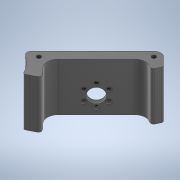
# Autodesk Inventor part: left_motor_short
Saved by Autodesk Inventor 2020 (Build 240168000, 168)
## iProperties
Created: 2023-12-16
Part Number: left_motor_short
Material: Пластмасса, непрозрачная, черная
Document SubType Name: Modeling
Designer: denis
Density: 0.952 g/cm^3
Appearance: Гладкая — черная
Author: denis
## iProperties of the stored document _3DПЕЧАТЬ.ipt
Created: 2024-02-21
Part Number: _3DПЕЧАТЬ
Material: Типовые
Document SubType Name: Modeling
Designer: 4s
Density: 1 g/cm^3
Appearance: По умолчанию
Author: 4s
Autodesk Inventor part; units mm, degrees
ref_plane "YZ Plane" through (0, 0, 0) normal (1, 0, 0) x (0, 1, 0)
ref_plane "XZ Plane" through (0, 0, 0) normal (0, 1, 0) x (-1, 0, 0)
ref_plane "XY Plane" through (0, 0, 0) normal (0, 0, 1) x (1, 0, 0)
sketch "Эскиз1" plane through (0, 0, 0) normal (0, 1, 0) x (-1, 0, 0)
  line L0 (34.2947, -76.014) -> (76.014, -34.2947)
  arc A0 (83.085, -34.2947) -> (76.014, -34.2947) centre (79.5495, -37.8302) ccw
  line L1 (83.085, -34.2947) -> (87.156, -38.3657)
  line L2 (46.3155, -73.8927) -> (73.8927, -46.3155)
  arc A1 (85.2064, -46.3155) -> (73.8927, -46.3155) centre (79.5495, -51.9723) ccw
  line L3 (85.2064, -46.3155) -> (87.5645, -48.6736)
  line L4 (92.5543, -49.5852) -> (94.5192, -45.7288)
  line L5 (87.156, -38.3657) -> (94.5192, -45.7288)
  line L6 (34.2947, -83.085) -> (38.3657, -87.156)
  arc A2 (34.2947, -76.014) -> (34.2947, -83.085) centre (37.8302, -79.5495) ccw
  arc A3 (46.3155, -73.8927) -> (46.3155, -85.2064) centre (51.9723, -79.5495) ccw
  line L7 (48.6736, -87.5645) -> (46.3155, -85.2064)
  line L8 (48.7014, -93.0224) -> (45.7288, -94.5192)
  line L9 (38.3657, -87.156) -> (45.7288, -94.5192)
  spline S0 degree 4 poles (87.5645, -48.6736) (88.1327, -49.2418) (88.8708, -49.8865) (89.7495, -50.471) (90.7127, -50.7263) (91.4939, -50.6999) (92.0261, -50.3682) (92.3519, -49.9478) (92.5543, -49.5852) knots 0 0 0 0 0 0.3763 0.501335 0.614666 0.722287 1 1 1 1 1
  spline S1 degree 4 poles (48.6736, -87.5645) (49.2196, -88.1111) (49.8318, -88.8375) (50.3553, -89.7359) (50.492, -90.7638) (50.3179, -91.6771) (49.7988, -92.3195) (49.2087, -92.7429) (48.7014, -93.0224) knots 0 0 0 0 0 0.349502 0.469309 0.582088 0.694155 1 1 1 1 1
  line L10 (-34.2947, -83.085) -> (-38.3657, -87.156)
  arc A4 (-34.2947, -83.085) -> (-34.2947, -76.014) centre (-37.8302, -79.5495) ccw
  line L11 (-34.2947, -76.014) -> (-76.014, -34.2947)
  arc A5 (-76.014, -34.2947) -> (-83.085, -34.2947) centre (-79.5495, -37.8302) ccw
  line L12 (-83.085, -34.2947) -> (-87.156, -38.3657)
  spline S2 degree 4 poles (-87.5645, -48.6736) (-88.2874, -48.92) (-89.2024, -49.1688) (-90.211, -49.3633) (-91.1746, -49.4987) (-91.8001, -49.5729) (-92.1944, -49.6036) (-92.4378, -49.611) (-92.5543, -49.5852) knots 0 0 0 0 0 0.417996 0.557878 0.680942 0.788351 1 1 1 1 1
  line L13 (-85.2064, -46.3155) -> (-87.5645, -48.6736)
  arc A6 (-73.8927, -46.3155) -> (-85.2064, -46.3155) centre (-79.5495, -51.9723) ccw
  line L14 (-46.3155, -73.8927) -> (-73.8927, -46.3155)
  arc A7 (-46.3155, -85.2064) -> (-46.3155, -73.8927) centre (-51.9723, -79.5495) ccw
  spline S3 degree 4 poles (-48.6736, -87.5645) (-49.2196, -88.1111) (-49.8318, -88.8375) (-50.3553, -89.7359) (-50.492, -90.7638) (-50.3179, -91.6771) (-49.7988, -92.3195) (-49.2087, -92.7429) (-48.7014, -93.0224) knots 0 0 0 0 0 0.349502 0.469309 0.582088 0.694155 1 1 1 1 1
  line L15 (-48.6736, -87.5645) -> (-46.3155, -85.2064)
  arc A8 (-92.5543, 49.5852) -> (-92.5543, -49.5852) centre (0, 0) ccw construction
  arc A9 (-48.7014, -93.0224) -> (48.7014, -93.0224) centre (0, 0) ccw construction
  line L16 (-38.3657, -87.156) -> (-45.7288, -94.5192)
  line L17 (-87.156, -38.3657) -> (-94.5192, -45.7288)
  line L18 (-92.5543, -49.5852) -> (-94.5192, -45.7288)
  line L19 (-48.7014, -93.0224) -> (-45.7288, -94.5192)
  line L20 (0, 0) -> (0, 95.3237) construction
  line L21 (34.2947, -76.014) -> (76.014, -34.2947)
  arc A10 (83.085, -34.2947) -> (76.014, -34.2947) centre (79.5495, -37.8302) ccw
  line L22 (83.085, -34.2947) -> (87.156, -38.3657)
  line L23 (46.3155, -73.8927) -> (73.8927, -46.3155)
  arc A11 (85.2064, -46.3155) -> (73.8927, -46.3155) centre (79.5495, -51.9723) ccw
  line L24 (85.2064, -46.3155) -> (87.5645, -48.6736)
  line L25 (92.5543, -49.5852) -> (94.5192, -45.7288)
  arc A12 (92.5543, -49.5852) -> (92.5543, 49.5852) centre (0, 0) ccw construction
  line L26 (87.156, -38.3657) -> (94.5192, -45.7288)
  line L27 (34.2947, -83.085) -> (38.3657, -87.156)
  arc A13 (34.2947, -76.014) -> (34.2947, -83.085) centre (37.8302, -79.5495) ccw
  arc A14 (46.3155, -73.8927) -> (46.3155, -85.2064) centre (51.9723, -79.5495) ccw
  line L28 (48.6736, -87.5645) -> (46.3155, -85.2064)
  line L29 (48.7014, -93.0224) -> (45.7288, -94.5192)
  line L30 (38.3657, -87.156) -> (45.7288, -94.5192)
  arc A15 (-48.7014, -93.0224) -> (48.7014, -93.0224) centre (0, 0) ccw construction
  spline S4 degree 4 poles (87.5645, -48.6736) (88.1327, -49.2418) (88.8708, -49.8865) (89.7495, -50.471) (90.7127, -50.7263) (91.4939, -50.6999) (92.0261, -50.3682) (92.3519, -49.9478) (92.5543, -49.5852) knots 0 0 0 0 0 0.3763 0.501335 0.614666 0.722287 1 1 1 1 1
  spline S5 degree 4 poles (48.6736, -87.5645) (49.2196, -88.1111) (49.8318, -88.8375) (50.3553, -89.7359) (50.492, -90.7638) (50.3179, -91.6771) (49.7988, -92.3195) (49.2087, -92.7429) (48.7014, -93.0224) knots 0 0 0 0 0 0.349502 0.469309 0.582088 0.694155 1 1 1 1 1
  line L31 (52.2091, 91.1) -> (48.6736, 87.5645) construction
  line L32 (52.2091, 91.1) -> (48.6736, 87.5645) construction
  line L33 (48.6736, 87.5645) -> (52.2091, 91.1) construction
  spline S6 degree 2 poles (48.6736, 87.5645) (52.2091, 91.1) (48.7014, 93.0224) knots 1 1 1 2 2 2 construction
  line L34 (52.2091, 91.1) -> (48.7014, 93.0224) construction
  line L35 (91.1, 52.2091) -> (52.2091, 91.1) construction
  arc A16 (92.5543, 49.5852) -> (48.7014, 93.0224) centre (0, 0) ccw construction
  line L36 (44.1942, 76.014) -> (76.014, 44.1942) construction
  line L37 (0, 56.6418) -> (-35.5516, 86.4744) construction
  arc A17 (0, 67.941) -> (23.7825, 76.5969) centre (0, 104.941) ccw construction
  arc A18 (-23.7825, 76.5969) -> (0, 67.941) centre (0, 104.941) ccw construction
  line L38 (-23.7825, 76.5969) -> (-35.2734, 86.2384) construction
  line L39 (0, 104.941) -> (-23.6028, 54.3247) construction
  arc A19 (-28.0199, 71.0163) -> (5.5413, 61.2914) centre (0, 104.941) ccw construction
  arc A20 (5.5413, 61.2914) -> (28.0199, 71.0163) centre (0, 104.941) ccw construction
  arc A21 (-30.6393, 73.2144) -> (-37.3889, 72.9198) centre (-33.8534, 69.3842) ccw construction
  line L40 (0, 56.6418) -> (23.7825, 76.5969) construction
  line L41 (23.7825, 76.5969) -> (35.2734, 86.2384) construction
  line L42 (0, 0) -> (74.2462, 74.2462) construction
  line L43 (42.6652, 95.941) -> (42.0492, 94.5734) construction
  line L44 (42.0492, 94.5734) -> (42.6652, 95.941) construction
  spline S7 degree 2 poles (42.0492, 94.5734) (42.6652, 95.941) (43.577, 95.5303) knots 1 1 1 2 2 2 construction
  line L45 (42.6652, 95.941) -> (43.577, 95.5303) construction
  arc A22 (-44.1942, 76.014) -> (-44.1942, 83.085) centre (-47.7297, 79.5495) ccw construction
  arc A23 (92.5543, -49.5852) -> (92.5543, 49.5852) centre (0, 0) ccw construction
  circle A24 centre (0, 0) radius 35 construction
  spline S8 degree 2 poles (-48.6736, 87.5645) (-52.2091, 91.1) (-48.7014, 93.0224) knots 1 1 1 2 2 2 construction
  line L46 (-48.6736, 87.5645) -> (-52.2091, 91.1) construction
  line L47 (-52.2091, 91.1) -> (-48.7014, 93.0224) construction
  arc A25 (-83.085, 44.1942) -> (-76.014, 44.1942) centre (-79.5495, 47.7297) ccw construction
  line L48 (-83.085, 44.1942) -> (-85.2064, 46.3155) construction
  line L49 (-44.1942, 76.014) -> (-46.3155, 73.8927) construction
  arc A26 (-48.7014, 93.0224) -> (-92.5543, 49.5852) centre (0, 0) ccw construction
  line L50 (-42.6652, 95.941) -> (-42.0492, 94.5734) construction
  arc A27 (-43.577, 95.5303) -> (-48.7014, 93.0224) centre (0, 0) ccw
  ellipse E0 centre (0, 102.7511) end of major axis (-44.5159, 105.2445) minor radius 28.887 (-42.0492, 94.5734) -> (-35.2734, 86.2384) ccw
  line L51 (-42.0492, 94.5734) -> (-42.6652, 95.941) construction
  spline S9 degree 2 poles (-42.0492, 94.5734) (-42.6652, 95.941) (-43.577, 95.5303) knots 1 1 1 2 2 2 construction
  line L52 (-42.6652, 95.941) -> (-43.577, 95.5303) construction
  line L53 (-42.0492, 94.5734) -> (-42.6652, 95.941) construction
  spline S10 degree 2 poles (-42.0492, 94.5734) (-42.6652, 95.941) (-43.577, 95.5303) knots 1 1 1 2 2 2
  line L54 (-42.6652, 95.941) -> (-43.577, 95.5303) construction
  line L55 (-42.6652, 95.941) -> (-43.577, 95.5303) construction
  line L56 (-44.1942, 83.085) -> (-48.6736, 87.5645) construction
  line L57 (-37.3889, 72.9198) -> (-76.014, 34.2947)
  arc A28 (-83.085, 34.2947) -> (-76.014, 34.2947) centre (-79.5495, 37.8302) ccw
  line L58 (-83.085, 34.2947) -> (-90.6891, 41.8987)
  arc A29 (-87.3563, 48.4654) -> (-90.6891, 41.8987) centre (0, 0) ccw construction
  line L59 (-93.5297, 47.6709) -> (-92.5543, 49.5852) construction
  arc A30 (85.2064, -46.3155) -> (73.8927, -46.3155) centre (79.5495, -51.9723) ccw construction
  line L60 (85.2064, -46.3155) -> (87.5645, -48.6736) construction
  spline S11 degree 2 poles (87.5645, -48.6736) (91.1, -52.2091) (92.5543, -49.5852) knots 1 1 1 2 2 2 construction
  line L61 (87.5645, -48.6736) -> (91.1, -52.2091) construction
  line L62 (91.1, -52.2091) -> (92.5543, -49.5852) construction
  line L63 (46.3155, -73.8927) -> (73.8927, -46.3155) construction
  line L64 (48.6736, -87.5645) -> (46.3155, -85.2064) construction
  line L65 (48.6736, -87.5645) -> (52.2091, -91.1) construction
  spline S12 degree 2 poles (48.6736, -87.5645) (52.2091, -91.1) (48.7014, -93.0224) knots 1 1 1 2 2 2 construction
  line L66 (52.2091, -91.1) -> (48.7014, -93.0224) construction
  arc A31 (46.3155, -73.8927) -> (46.3155, -85.2064) centre (51.9723, -79.5495) ccw construction
  arc A32 (48.7014, -93.0224) -> (92.5543, -49.5852) centre (0, 0) ccw construction
  arc A33 (-48.7014, -93.0224) -> (48.7014, -93.0224) centre (0, 0) ccw construction
  arc A34 (-90.6891, 41.8987) -> (-87.3563, 48.4654) centre (0, 0) ccw construction
  line L67 (42.6652, 95.941) -> (-42.6652, 95.941) construction
  line L68 (-48.6736, -87.5645) -> (-52.2091, -91.1) construction
  spline S13 degree 2 poles (-48.6736, -87.5645) (-52.2091, -91.1) (-48.7014, -93.0224) knots 1 1 1 2 2 2 construction
  line L69 (-52.2091, -91.1) -> (-48.7014, -93.0224) construction
  line L70 (-91.1, -52.2091) -> (-92.5543, -49.5852) construction
  spline S14 degree 2 poles (-87.5645, -48.6736) (-91.1, -52.2091) (-92.5543, -49.5852) knots 1 1 1 2 2 2 construction
  line L71 (-87.5645, -48.6736) -> (-91.1, -52.2091) construction
  arc A35 (-92.5543, -49.5852) -> (-48.7014, -93.0224) centre (0, 0) ccw construction
  line L72 (-48.6736, -87.5645) -> (-46.3155, -85.2064) construction
  arc A36 (-73.8927, -46.3155) -> (-85.2064, -46.3155) centre (-79.5495, -51.9723) ccw construction
  line L73 (-85.2064, -46.3155) -> (-87.5645, -48.6736) construction
  line L74 (-46.3155, -73.8927) -> (-73.8927, -46.3155) construction
  arc A37 (-46.3155, -85.2064) -> (-46.3155, -73.8927) centre (-51.9723, -79.5495) ccw construction
  arc A38 (-92.5543, 49.5852) -> (-92.5543, -49.5852) centre (0, 0) ccw construction
  arc A39 (44.1942, 83.085) -> (44.1942, 76.014) centre (47.7297, 79.5495) ccw construction
  arc A40 (44.0271, 95.3237) -> (43.577, 95.5303) centre (0, 0) ccw construction
  line L75 (42.6652, 95.941) -> (43.577, 95.5303) construction
  arc A41 (48.7014, 93.0224) -> (44.0271, 95.3237) centre (0, 0) ccw construction
  line L76 (52.2091, 91.1) -> (48.7014, 93.0224) construction
  line L77 (83.085, 44.1942) -> (87.5645, 48.6736) construction
  ellipse E1 centre (0, 102.7511) end of major axis (44.5159, 105.2445) minor radius 28.887 (35.2734, 86.2384) -> (42.0492, 94.5734) ccw construction
  arc A42 (76.014, 44.1942) -> (83.085, 44.1942) centre (79.5495, 47.7297) ccw construction
  line L78 (0, 0) -> (0, 209.8821) construction
  arc A43 (43.577, 95.5303) -> (-43.577, 95.5303) centre (0, 0) ccw construction
  arc A44 (23.7825, 76.5969) -> (0, 67.941) centre (0, 104.941) ccw construction
  line L79 (44.0271, 95.3237) -> (44.0271, 127.8162) construction
  ellipse E2 centre (0, 102.7511) end of major axis (44.0271, 102.7511) minor radius 27.5932 (42.0492, 94.5734) -> (35.2734, 86.2384) ccw construction
  line L80 (-30.6393, 73.2144) -> (-28.0199, 71.0163) construction
  arc A45 (28.0199, 71.0163) -> (-28.0199, 71.0163) centre (0, 104.941) ccw construction
  line L81 (30.6393, 73.2144) -> (28.0199, 71.0163) construction
  arc A46 (37.3889, 72.9198) -> (30.6393, 73.2144) centre (33.8534, 69.3842) ccw construction
  line L82 (44.0271, 95.3237) -> (43.577, 95.5303) construction
  arc A47 (44.1942, 83.085) -> (44.1942, 76.014) centre (47.7297, 79.5495) ccw construction
  line L83 (48.6736, 87.5645) -> (44.1942, 83.085) construction
  line L84 (37.3889, 72.9198) -> (76.014, 34.2947) construction
  line L85 (44.1942, 76.014) -> (76.014, 44.1942) construction
  arc A48 (76.014, 44.1942) -> (83.085, 44.1942) centre (79.5495, 47.7297) ccw construction
  arc A49 (76.014, 34.2947) -> (83.085, 34.2947) centre (79.5495, 37.8302) ccw construction
  line L86 (83.085, 44.1942) -> (87.3563, 48.4654) construction
  line L87 (83.085, 34.2947) -> (90.6891, 41.8987) construction
  arc A50 (90.6891, 41.8987) -> (87.3563, 48.4654) centre (0, 0) ccw construction
  arc A51 (-83.085, 34.2947) -> (-76.014, 34.2947) centre (-79.5495, 37.8302) ccw
  line L88 (-87.156, 38.3657) -> (-94.5192, 45.7288)
  line L89 (-93.0224, 48.7014) -> (-94.5192, 45.7288)
  arc A52 (-85.2064, 46.3155) -> (-73.8927, 46.3155) centre (-79.5495, 51.9723) ccw
  line L90 (-87.5645, 48.6736) -> (-85.2064, 46.3155)
  line L91 (-83.085, 34.2947) -> (-87.156, 38.3657)
  line L92 (-73.8927, 46.3155) -> (-46.3155, 73.8927)
  spline S15 degree 4 poles (-87.5645, 48.6736) (-88.1111, 49.2196) (-88.8375, 49.8318) (-89.7359, 50.3553) (-90.7638, 50.492) (-91.6771, 50.3179) (-92.3195, 49.7988) (-92.7429, 49.2087) (-93.0224, 48.7014) knots 0 0 0 0 0 0.349502 0.469309 0.582088 0.694155 1 1 1 1 1
  arc A53 (-34.2947, 76.014) -> (-34.2947, 83.085) centre (-37.8302, 79.5495) ccw construction
  line L93 (-34.2947, 83.085) -> (-38.3657, 87.156) construction
  arc A54 (-46.3155, 73.8927) -> (-46.3155, 85.2064) centre (-51.9723, 79.5495) ccw
  line L94 (-46.3155, 85.2064) -> (-48.6736, 87.5645)
  spline S16 degree 4 poles (-48.6736, 87.5645) (-49.2418, 88.1327) (-49.8865, 88.8708) (-50.471, 89.7495) (-50.7263, 90.7127) (-50.6999, 91.4939) (-50.3682, 92.0261) (-49.9478, 92.3519) (-49.5852, 92.5543) knots 0 0 0 0 0 0.3763 0.501335 0.614666 0.722287 1 1 1 1 1
  line L95 (-49.5852, 92.5543) -> (-45.7288, 94.5192)
  line L96 (-38.3657, 87.156) -> (-45.7288, 94.5192) construction
  arc A55 (-34.2947, 76.014) -> (-34.2947, 83.085) centre (-37.8302, 79.5495) ccw construction
  line L97 (-34.2947, 83.085) -> (-38.3657, 87.156) construction
  arc A56 (-46.3155, 73.8927) -> (-46.3155, 85.2064) centre (-51.9723, 79.5495) ccw
  line L98 (-46.3155, 85.2064) -> (-48.6736, 87.5645)
  spline S17 degree 4 poles (-48.6736, 87.5645) (-49.2418, 88.1327) (-49.8865, 88.8708) (-50.471, 89.7495) (-50.7263, 90.7127) (-50.6999, 91.4939) (-50.3682, 92.0261) (-49.9478, 92.3519) (-49.5852, 92.5543) knots 0 0 0 0 0 0.3763 0.501335 0.614666 0.722287 1 1 1 1 1
  line L99 (-49.5852, 92.5543) -> (-45.7288, 94.5192)
  line L100 (-38.3657, 87.156) -> (-45.7288, 94.5192) construction
  arc A57 (-83.085, 34.2947) -> (-76.014, 34.2947) centre (-79.5495, 37.8302) ccw
  line L101 (-83.085, 34.2947) -> (-87.156, 38.3657)
  line L102 (-87.156, 38.3657) -> (-94.5192, 45.7288)
  line L103 (-93.0224, 48.7014) -> (-94.5192, 45.7288)
  spline S18 degree 4 poles (-87.5645, 48.6736) (-88.1111, 49.2196) (-88.8375, 49.8318) (-89.7359, 50.3553) (-90.7638, 50.492) (-91.6771, 50.3179) (-92.3195, 49.7988) (-92.7429, 49.2087) (-93.0224, 48.7014) knots 0 0 0 0 0 0.349502 0.469309 0.582088 0.694155 1 1 1 1 1
  arc A58 (-85.2064, 46.3155) -> (-73.8927, 46.3155) centre (-79.5495, 51.9723) ccw
  line L104 (-76.014, 34.2947) -> (-34.2947, 76.014) construction
  line L105 (-73.8927, 46.3155) -> (-46.3155, 73.8927)
  line L106 (-87.5645, 48.6736) -> (-85.2064, 46.3155)
  line L107 (-87.5645, 48.6736) -> (-91.1, 52.2091) construction
  spline S19 degree 2 poles (-87.5645, 48.6736) (-91.1, 52.2091) (-93.0224, 48.7014) knots 1 1 1 2 2 2 construction
  line L108 (-91.1, 52.2091) -> (-93.0224, 48.7014) construction
  line L109 (-48.6736, 87.5645) -> (-52.2091, 91.1) construction
  spline S20 degree 2 poles (-48.6736, 87.5645) (-52.2091, 91.1) (-49.5852, 92.5543) knots 1 1 1 2 2 2 construction
  line L110 (-52.2091, 91.1) -> (-49.5852, 92.5543) construction
  arc A59 (-49.5852, 92.5543) -> (-93.0224, 48.7014) centre (0, 0) ccw construction
  arc A60 (-46.3155, 73.8927) -> (-46.3155, 85.2064) centre (-51.9723, 79.5495) ccw construction
  line L111 (-46.3155, 85.2064) -> (-48.6736, 87.5645) construction
  line L112 (-73.8927, 46.3155) -> (-46.3155, 73.8927) construction
  arc A61 (-85.2064, 46.3155) -> (-73.8927, 46.3155) centre (-79.5495, 51.9723) ccw construction
  line L113 (-87.5645, 48.6736) -> (-85.2064, 46.3155) construction
  line L114 (-60.1041, 60.1041) -> (-55.1543, 55.1543) construction
  circle A62 centre (-79.5495, 37.8302) radius 1.5
  circle A63 centre (-37.8302, 79.5495) radius 1.5
  arc A64 (-34.995, 78.2699) -> (-31.4954, 78.8132) centre (-33.6167, 80.9346) ccw construction
  arc A65 (-36.5845, 80.4956) -> (-34.995, 78.2699) centre (-33.6167, 80.9346) ccw construction
  arc A66 (-31.7687, 83.2978) -> (-36.5845, 80.4956) centre (-33.6167, 80.9346) ccw construction
  arc A67 (-31.4954, 78.8132) -> (-31.7687, 83.2978) centre (-33.6167, 80.9346) ccw
  line L115 (-31.4954, 78.8132) -> (-29.1816, 81.127) construction
  line L116 (-46.3155, 73.8927) -> (-73.8927, 46.3155)
  line L117 (-73.8927, 46.3155) -> (-76.014, 44.1942) construction
  line L118 (-85.2064, 46.3155) -> (-87.3563, 48.4654)
  line L119 (-31.7687, 83.2978) -> (-35.2734, 86.2384)
  line L120 (99.9, 0) -> (-99.9, 0) construction
  line L121 (-31.4954, 78.8132) -> (-37.3889, 72.9198)
  point P0 (49.5385, -88.5397)
  point P1 (50.0866, -89.3893)
  point P2 (50.374, -90.1304)
  point P3 (50.4468, -90.7861)
  point P4 (50.3313, -91.3833)
  point P5 (50.0252, -91.9468)
  point P6 (49.4982, -92.4922)
  point P7 (88.5759, -49.5937)
  point P8 (89.4338, -50.2024)
  point P9 (90.1559, -50.5529)
  point P10 (90.7644, -50.6948)
  point P11 (91.2858, -50.6665)
  point P12 (91.7467, -50.4838)
  point P13 (92.1672, -50.1352)
  point P14 (-49.5385, -88.5397)
  point P15 (-50.0866, -89.3893)
  point P16 (-50.374, -90.1304)
  point P17 (-50.4468, -90.7861)
  point P18 (-50.3313, -91.3833)
  point P19 (-50.0252, -91.9468)
  point P20 (-49.4982, -92.4922)
  point P21 (-88.8035, -49.0449)
  point P22 (-89.8171, -49.2759)
  point P23 (-90.6238, -49.4176)
  point P24 (-91.2517, -49.506)
  point P25 (-91.7347, -49.5616)
  point P26 (-92.1038, -49.5932)
  point P27 (-92.3767, -49.6023)
  point P28 (88.5759, -49.5937)
  point P29 (89.4338, -50.2024)
  point P30 (90.1559, -50.5529)
  point P31 (90.7644, -50.6948)
  point P32 (91.2858, -50.6665)
  point P33 (91.7467, -50.4838)
  point P34 (92.1672, -50.1352)
  point P35 (49.5385, -88.5397)
  point P36 (50.0866, -89.3893)
  point P37 (50.374, -90.1304)
  point P38 (50.4468, -90.7861)
  point P39 (50.3313, -91.3833)
  point P40 (50.0252, -91.9468)
  point P41 (49.4982, -92.4922)
  point P42 (79.5495, 40.6586)
  point P43 (40.6586, 79.5495)
  point P44 (60.1041, 60.1041)
  point P45 (-23.542, 76.3968)
  point P46 (-34.9935, 86.0061)
  point P47 (0, 95.941)
  point P48 (-15.6369, 71.4076)
  point P49 (-13.2817, 58.6489)
  point P50 (-28.5452, 71.4571)
  point P51 (13.2817, 58.6489)
  point P52 (-87.5645, 48.6736)
  point P53 (0, 105)
  point P54 (-94.5192, 45.7288)
  point P55 (0, 95.941)
  point P56 (-88.5397, 49.5385)
  point P57 (-89.3893, 50.0866)
  point P58 (-90.1304, 50.374)
  point P59 (-90.7861, 50.4468)
  point P60 (-91.3833, 50.3313)
  point P61 (-91.9468, 50.0252)
  point P62 (-92.4922, 49.4982)
  point P63 (-49.5937, 88.5759)
  point P64 (-50.2024, 89.4338)
  point P65 (-50.5529, 90.1559)
  point P66 (-50.6948, 90.7644)
  point P67 (-50.6665, 91.2858)
  point P68 (-50.4838, 91.7467)
  point P69 (-50.1352, 92.1672)
  point P70 (-49.5937, 88.5759)
  point P71 (-50.2024, 89.4338)
  point P72 (-50.5529, 90.1559)
  point P73 (-50.6948, 90.7644)
  point P74 (-50.6665, 91.2858)
  point P75 (-50.4838, 91.7467)
  point P76 (-50.1352, 92.1672)
  point P77 (-88.5397, 49.5385)
  point P78 (-89.3893, 50.0866)
  point P79 (-90.1304, 50.374)
  point P80 (-90.7861, 50.4468)
  point P81 (-91.3833, 50.3313)
  point P82 (-91.9468, 50.0252)
  point P83 (-92.4922, 49.4982)
  dimension "d63" = 44.5856
  dimension "d44" = 74
  dimension "d45" = 100
  dimension "d46" = 28
  dimension "d47" = 15
  dimension "d48" = 45
  dimension "d49" = 55
  dimension "d50" = 16.3348
  dimension "d51" = 27.5
  dimension "d52" = 5
  dimension "d53" = 5
  dimension "d54" = 1
  dimension "d55" = 1.5
  dimension "d56" = 1.5
  dimension "d57" = 1
  dimension "d58" = 4
  dimension "d59" = 70
  dimension "d60" = 85
  dimension "d61" = 105
  dimension "d62" = 1.3619
  dimension "d64" = 88
  dimension "d65" = 7
  dimension "d66" = 5
  dimension "d67" = 7
  dimension "d68" = 5
  dimension "d69" = 7
  dimension "d70" = 5
  dimension "d71" = 5.1
  dimension "d72" = 3
  dimension "d73" = 6
  constraints: 200 end point, 159 point on circle, 145 symmetric about line, 67 centre point, 28 coincident, 20 point on line, 18 tangent, 11 collinear, 8 parallel, 6 midpoint, 4 vertical, 3 perpendicular, 2 horizontal, 1 concentric, 1 equal radius, 182 other
  measures "d44" diameter of A44
  measures "d45" angle of L37 L40
  measures "d46" distance from line of L67 A18.end
  measures "d47" distance of L40.end L41.end
  measures "d48" angle of L78 L42
  measures "d49" distance of point (40.659, 79.55) point (79.55, 40.659)
  measures "d50" distance of L35.start point (79.55, 40.659)
  measures "d51" distance of point (40.659, 79.55) point (60.104, 60.104)
  measures "d52" radius of A39
  measures "d53" distance of L76.start L31.end
  measures "d54" distance of L43.start L45.end
  measures "d55" distance of L43.start L43.end
  measures "d56" distance of L55.start L51.start
  measures "d57" distance of L55.start L52.end
  measures "d58" distance of L76.start L34.end
  measures "d59" diameter of A24
  measures "d60" distance of point (60.104, 60.104) L78.start
  measures "d61" radius of A23
  measures "d62" distance from line of L79 L67.start
  measures "d64" diameter of A45
  measures "d65" distance between parallel lines of L48 L58
  measures "d66" radius of A25
  measures "d67" distance between parallel lines of L57 L49
  measures "d68" radius of A28
  measures "d69" distance between parallel lines of L37 L80
  measures "d70" radius of A21
  measures "d71" radial gap between concentric circles of A38 A34
  measures "d72" diameter of A62
  measures "d73" diameter of A64
extrude "Выдавливание10" add sketch "Эскиз1" along normal blind 35 contours S10 E0 L119 A67 L121 L57 A28 L58 L88 L89 S15 L90 A52 L92 A54 L94 S16 L95 A27
sketch "Эскиз6" plane through (31.4954, 0, 78.8132) normal (-0.7071, 0, -0.7071) x (-0.7071, 0, 0.7071)
  line L0 (-5.4588, 35) -> (-2.4588, 35) construction
  line L1 (-64.4588, 35) -> (-61.4588, 35) construction
  line L2 (-61.4588, 0) -> (-64.4588, 0) construction
  line L3 (-5.8588, 0) -> (-2.0588, 0) construction
  line L4 (-62.9588, 0) -> (-67.9588, 0) construction
  line L5 (-62.9588, 35) -> (-62.9588, 0) construction
  line L6 (-62.9588, 35) -> (0, 35) construction
  line L7 (-121.9588, 35) -> (-121.9588, 0) construction
  line L8 (-62.9588, 0) -> (0, 0) construction
  circle A0 centre (-33.4588, 12) radius 10.65
  circle A1 centre (-33.4588, 12) radius 7.5 construction
  circle A2 centre (-33.4588, 12) radius 5.2
  circle A3 centre (-33.4588, 19.5) radius 1.25
  line L9 (-33.4588, 12) -> (-33.4588, 35) construction
  line L10 (-13.9588, 35) -> (-52.9588, 35) construction
  circle A4 centre (-39.9539, 15.75) radius 1.25
  circle A5 centre (-39.9539, 8.25) radius 1.25
  circle A6 centre (-33.4588, 4.5) radius 1.25
  circle A7 centre (-26.9636, 8.25) radius 1.25
  circle A8 centre (-26.9636, 15.75) radius 1.25
  point P0 (-33.4588, 0)
  dimension "d82" = 15
  dimension "d80" = 59
  dimension "d81" = 21.3
  dimension "d83" = 10.4
  dimension "d84" = 2.5
  dimension "d87" = 360
  dimension "d96" = 12
  constraints: 8 centre point, 6 end point, 3 point on line, 2 coincident, 2 midpoint, 2 perpendicular, 1 vertical, 1 vertical alignment, 15 other
  measures "d80" distance between parallel lines of L7 L5
  measures "d81" diameter of A0
  measures "d83" diameter of A2
  measures "d84" diameter of A3
  measures "d96" distance from line of L8 A0.centre
extrude "Выдавливание13" cut sketch "Эскиз6" against normal mid plane 33.5 contours A2 | A3 | A4 | A5 | A6 | A7 | A8
extrude "Выдавливание14" cut sketch "Эскиз6" against normal blind 3.5
chamfer "Фаска3" distance 0.5 angle 45 6 edges at (60.988, 19.5, 59.2202) (65.5808, 15.75, 54.6274) (65.5808, 8.25, 54.6274) (60.988, 4.5, 59.2202) (56.3952, 8.25, 63.813) (56.3952, 15.75, 63.813)
sketch "Эскиз7" plane through (0, 35, 0) normal (0, 1, 0) x (1, 0, 0)
  circle A0 centre (0, 0) radius 98
  line L0 (83.394, -51.4727) -> (105.1705, -56.0334)
  line L1 (105.1705, -56.0334) -> (91.253, -35.7336)
  dimension "d97" = 196
  constraints: 4 end point, 2 point on circle, 1 centre point, 1 coincident
  measures "d97" diameter of A0
extrude "Выдавливание15" cut sketch "Эскиз7" against normal blind 41.5 contours A0 L1 L0
fillet "Сопряжение1" radius 2 2 edges at (85.9577, 17.5, 47.0668) (89.2556, 17.5, 40.4652)
